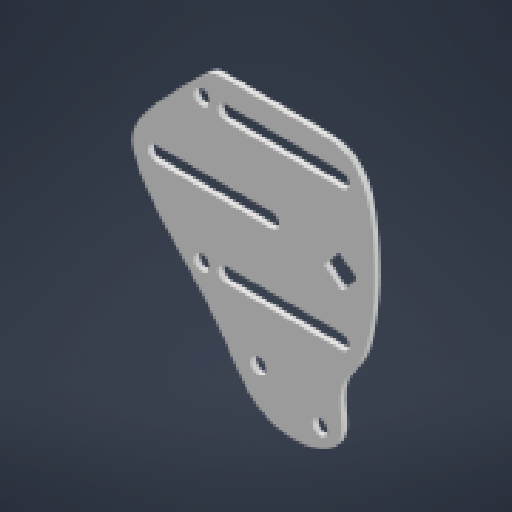
# Autodesk Inventor part: tracking-wheel-mount-v2
Saved by Autodesk Inventor 2023.2 (Build 272271000, 271)
## iProperties
Created: 2023-03-27
Part Number: tracking-wheel-mount-v2
Material: Generic
Document SubType Name: Modeling
Designer: Liam
Density: 1 g/cm^3
Appearance: Default
Author: Liam
Autodesk Inventor part; units mm, degrees
ref_plane "YZ Plane" through (0, 0, 0) normal (1, 0, 0) x (0, 1, 0)
ref_plane "XZ Plane" through (0, 0, 0) normal (0, 1, 0) x (-1, 0, 0)
ref_plane "XY Plane" through (0, 0, 0) normal (0, 0, 1) x (1, 0, 0)
sketch "Sketch1" plane through (0, 0, 0) normal (0, 0, 1) x (1, 0, 0)
  line L0 (-1.5875, -283.7942) -> (-33.3375, -283.7942)
  line L1 (-1.5875, -287.7058) -> (-33.3375, -287.7058)
  arc A0 (-33.3375, -283.7942) -> (-33.3375, -287.7058) centre (-33.3375, -285.75) ccw
  arc A1 (-1.5875, -287.7058) -> (-1.5875, -283.7942) centre (-1.5875, -285.75) ccw
  line L2 (17.4625, -264.7442) -> (-14.2875, -264.7442)
  line L3 (17.4625, -268.6558) -> (-14.2875, -268.6558)
  arc A2 (-14.2875, -264.7442) -> (-14.2875, -268.6558) centre (-14.2875, -266.7) ccw
  arc A3 (17.4625, -268.6558) -> (17.4625, -264.7442) centre (17.4625, -266.7) ccw
  arc A4 (17.4625, -306.7558) -> (17.4625, -302.8442) centre (17.4625, -304.8) ccw
  line L4 (17.4625, -306.7558) -> (-14.2875, -306.7558)
  arc A5 (-14.2875, -302.8442) -> (-14.2875, -306.7558) centre (-14.2875, -304.8) ccw
  line L5 (17.4625, -302.8442) -> (-14.2875, -302.8442)
  line L6 (-1.5875, -285.75) -> (-33.3375, -285.75)
  line L7 (-39.6875, -285.75) -> (-39.6875, -281.3199) construction
  line L8 (-39.6875, -281.3199) -> (-31.1834, -271.3984) construction
  line L9 (-31.1834, -271.3984) -> (-18.9197, -259.2751) construction
  line L10 (-18.9197, -259.2751) -> (-17.4625, -258.7024) construction
  line L11 (-17.4625, -258.7024) -> (-13.3504, -258.7024) construction
  line L12 (-13.3504, -258.7024) -> (-9.7175, -258.7024) construction
  line L13 (-9.7175, -258.7024) -> (-3.3988, -258.7024) construction
  line L14 (-3.3988, -258.7024) -> (0.4625, -258.7024) construction
  line L15 (0.4625, -258.7024) -> (15.1943, -258.7024) construction
  line L16 (15.1943, -258.7024) -> (17.4625, -258.7024) construction
  line L17 (17.4625, -258.7024) -> (26.4353, -264.5027) construction
  line L18 (26.4353, -264.5027) -> (26.4353, -285.75) construction
  spline S0 degree 4 poles (-39.6875, -285.75) (-39.6875, -281.3199) (-31.1834, -271.3984) (-18.9197, -259.2751) (-17.4625, -258.7024) (-13.3504, -258.7024) (-9.7175, -258.7024) (-3.3988, -258.7024) (0.4625, -258.7024) (15.1943, -258.7024) (17.4625, -258.7024) (26.4353, -264.5027) (26.4353, -285.75) knots 1 1 1 1 1 2 3 4 5 6 7 8 9 10 10 10 10 10
  line L19 (20.9977, -287.5498) -> (17.0087, -284.4043)
  arc A6 (21.1032, -288.4416) -> (20.9977, -287.5498) centre (20.6045, -288.0484) ccw
  line L20 (17.9577, -292.4306) -> (21.1032, -288.4416)
  arc A7 (17.0659, -292.5361) -> (17.9577, -292.4306) centre (17.4591, -292.0375) ccw
  line L21 (13.0768, -289.3906) -> (17.0659, -292.5361)
  arc A8 (12.9714, -288.4988) -> (13.0768, -289.3906) centre (13.47, -288.892) ccw
  line L22 (16.1169, -284.5098) -> (12.9714, -288.4988)
  arc A9 (17.0087, -284.4043) -> (16.1169, -284.5098) centre (16.6155, -284.9029) ccw
  circle A10 centre (-20.6084, -305.2253) radius 2.0955
  circle A11 centre (-20.6084, -266.2747) radius 2.0955
  circle A12 centre (11.5295, -327.8898) radius 2.0955
  line L23 (-39.6875, -285.75) -> (-39.6875, -288.4988) construction
  line L24 (-39.6875, -288.4988) -> (-35.4355, -296.4735) construction
  line L25 (-35.4355, -296.4735) -> (-28.6542, -303.7638) construction
  line L26 (-28.6542, -303.7638) -> (-22.7039, -309.9306) construction
  line L27 (-22.7039, -309.9306) -> (-15.6661, -317.7268) construction
  line L28 (-15.6661, -317.7268) -> (-9.739, -328.1678) construction
  line L29 (-9.739, -328.1678) -> (-3.3988, -334.115) construction
  line L30 (-3.3988, -334.115) -> (8.8016, -335.3618) construction
  line L31 (8.8016, -335.3618) -> (20.2246, -329.5087) construction
  line L32 (20.2246, -329.5087) -> (15.3145, -317.7268) construction
  line L33 (15.3145, -317.7268) -> (19.5304, -310.4349) construction
  line L34 (19.5304, -310.4349) -> (24.1196, -307.3208) construction
  line L35 (24.1196, -307.3208) -> (26.4353, -292.0468) construction
  line L36 (26.4353, -292.0468) -> (26.4353, -285.75) construction
  spline S1 degree 4 poles (-39.6875, -285.75) (-39.6875, -288.4988) (-35.4355, -296.4735) (-28.6542, -303.7638) (-22.7039, -309.9306) (-15.6661, -317.7268) (-9.739, -328.1678) (-3.3988, -334.115) (8.8016, -335.3618) (20.2246, -329.5087) (15.3145, -317.7268) (19.5304, -310.4349) (24.1196, -307.3208) (26.4353, -292.0468) (26.4353, -285.75) knots 1 1 1 1 1 2 3 4 5 6 7 8 9 10 11 12 12 12 12 12
  circle A13 centre (-5.245, -321.8562) radius 2.0955
  point P0 (0, 0)
  point P1 (-7.9375, -285.75)
  point P2 (11.1125, -266.7)
  point P3 (11.1125, -304.8)
  point P4 (19.4183, -304.8)
  dimension "d0" = 31.75
  dimension "d3" = 0
  dimension "d4" = 3.9116
  dimension "d5" = 0
  dimension "d8" = 3.9116
  dimension "d9" = 0
  dimension "d10" = 31.75
  dimension "d11" = 0
  dimension "d12" = 6.35
  dimension "d13" = 6.35
  dimension "d14" = 3.9116
  dimension "d15" = 0
  dimension "d16" = 31.75
  dimension "d19" = 0
  dimension "d20" = 6.35
  dimension "d57" = 6.35
  dimension "d58" = 0
  dimension "d60" = 0
  dimension "d61" = 7.017
  dimension "d64" = 4.191
  dimension "d67" = 4.191
  dimension "d70" = 4.191
  dimension "d73" = 4.191
  constraints: 22 end point, 21 point on circle, 14 centre point, 6 horizontal, 6 tangent, 4 parallel, 4 vertical, 20 other
  measures "d0" distance of L6.start L6.end
  measures "d3" vertical distance of point (-7.937, -285.75) L6.start
  measures "d4" distance between parallel lines of L0 L1
  measures "d5" horizontal distance of L0.start L1.start
  measures "d8" distance between parallel lines of L2 L3
  measures "d9" horizontal distance of L2.start L3.start
  measures "d10" distance of L3.start L3.end
  measures "d11" vertical distance of point (11.113, -266.7) A3.centre
  measures "d12" distance of L6.start point (-7.937, -285.75)
  measures "d13" distance of A3.centre point (11.113, -266.7)
  measures "d14" distance between parallel lines of L5 L4
  measures "d15" horizontal distance of L5.start L4.start
  measures "d16" distance of L4.start L4.end
  measures "d19" vertical distance of point (11.113, -304.8) A4.centre
  measures "d20" distance of point (11.113, -304.8) A4.centre
  measures "d57" distance of L6.end L7.start
  measures "d58" vertical distance of L6.end L7.start
  measures "d60" vertical distance of L6.start L18.end
  measures "d61" horizontal distance of point (19.418, -304.8) L18.end
  measures "d64" diameter of A10
  measures "d67" diameter of A11
  measures "d70" diameter of A12
  measures "d73" diameter of A13
extrude "Extrusion3" add sketch "Sketch1" against normal blind 1.524
equation "\"d8\" = d4"
equation "\"d10\" = d0"
equation "\"d13\" = d12"
equation "\"d14\" = d4"
equation "\"d16\" = d0"
equation "\"d20\" = d12"
body "Solid3"
